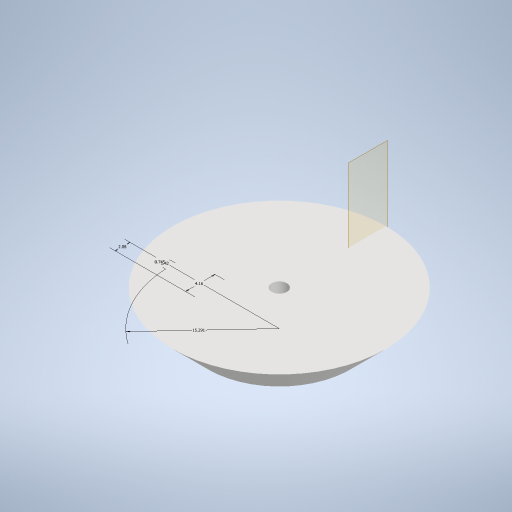
# Autodesk Inventor part: bevelGear
Saved by Autodesk Inventor 2023 (Build 270158000, 158)
## iProperties
Created: 2022-11-18
Part Number: bevelGear
Material: Generic
Document SubType Name: Modeling
Designer: shrey
Density: 1 g/cm^3
Appearance: Default
Author: shrey
Autodesk Inventor part; units mm, degrees
ref_plane "YZ Plane" through (0, 0, 0) normal (1, 0, 0) x (0, 1, 0)
ref_plane "XZ Plane" through (0, 0, 0) normal (0, 1, 0) x (-1, 0, 0)
ref_plane "XY Plane" through (0, 0, 0) normal (0, 0, 1) x (1, 0, 0)
ref_plane "Work Plane1" through (0, 0, 0) normal (1, 0, 0) x (0, 1, 0)
sketch "Sketch1" plane through (0, 0, 0) normal (1, 0, 0) x (0, 1, 0)
  line L0 (0, 0) -> (5, 0) construction
  line L1 (5, 0) -> (5, 5)
  line L2 (0, 5) -> (0, 0) construction
  line L3 (0, 5) -> (5, 0)
  line L4 (0, 5) -> (5, 5)
  line L5 (5, 0) -> (0, 0) construction
  line L6 (0, 0) -> (0, 30)
  line L7 (0, 30) -> (5, 30) construction
  line L8 (5, 30) -> (5, 0)
  line L9 (0, 30) -> (5, 30)
  line L10 (5, 30) -> (5, 25)
  line L11 (5, 25) -> (0, 25)
  line L12 (0, 25) -> (0, 30)
  line L13 (0, 25) -> (5, 30)
  line L14 (0, 15) -> (5, 15) construction
  line L15 (0, 13.925) -> (5, 13.925)
  line L16 (5, 13.925) -> (5, 16.075)
  line L17 (5, 16.075) -> (0, 16.075)
  line L18 (0, 16.075) -> (0, 13.925)
  point P0 (10, 5)
  point P1 (0, 16.075)
  point P2 (0, 25)
  dimension "d4" = 5
  dimension "d10" = 30
  dimension "d11" = 5
  dimension "d12" = 5
  dimension "d13" = 5
  dimension "d14" = 5
  dimension "d15" = 1.075
  dimension "d16" = 2.15
  constraints: 38 end point, 7 parallel, 5 horizontal, 4 perpendicular, 2 midpoint, 2 point on line
  measures "d4" distance of L1.end L0.end
  measures "d10" distance of L5.end L6.end
  measures "d11" distance of L6.end L7.end
  measures "d12" distance of L2.start L4.end
  measures "d13" distance of L10.end L11.end
  measures "d14" distance of L9.end L10.end
  measures "d15" distance between parallel lines of L14 L17
  measures "d16" distance between parallel lines of L15 L17
revolve "Revolution1" add sketch "Sketch1" angle 360 about axis through (0, 0, 15) along (0, 1, 0) contours L3 L4 L1 | L4 L6 L15 L8 | L17 L6 L11 L8 | L11 L13 L8
sketch "Sketch2" plane through (0, 0, 15) normal (0, -1, 0) x (1, 0, 0)
  arc A0 (0, 1.075) -> (0, -1.075) centre (0, 0) ccw projected
  arc A1 (0, 10) -> (0, -10) centre (0, 0) ccw construction
  arc A2 (-9.7813, 2.08) -> (-9.7813, -2.08) centre (0, 0) ccw
  arc A3 (-15.2728, 0.745) -> (-15.2761, -0.675) centre (0, 0) ccw
  point P0 (0, -15)
  dimension "d17" = 4.16
  dimension "d18" = 2.08
  dimension "d21" = 0.745
  dimension "d22" = 1.42
  dimension "d23" = 15.291
  constraints: 6 point on circle, 2 centre point, 2 coincident
  measures "d17" distance of A2.start A2.end
  measures "d18" vertical distance of A2.centre A2.start
  measures "d21" vertical distance of A2.centre A3.start
  measures "d22" distance of A3.start A3.end
  measures "d23" radius of A3
equation "\"t\" = 0.15"
